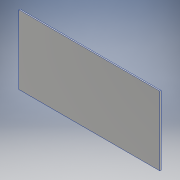
# Autodesk Inventor part: Led Plater
Saved by Autodesk Inventor 2017 (Build 210142000, 142)
## iProperties
Created: 2017-01-06
Part Number: Led Plater
Material: Aluminum 6061
Document SubType Name: Modeling
Designer: umr
Density: 2.7 g/cm^3
Appearance: Aluminum - Flat
Author: umr
Autodesk Inventor part; units mm, degrees
ref_plane "YZ Plane" through (0, 0, 0) normal (1, 0, 0) x (0, 1, 0)
sketch "Sketch1" plane through (0, 0, 0) normal (0, 1, 0) x (-1, 0, 0)
  line L0 (0, 0) -> (2550, 0)
  line L1 (2550, 0) -> (2550, -1250)
  line L2 (2550, -1250) -> (0, -1250)
  line L3 (0, -1250) -> (0, 0)
  dimension "d0" = 1250
  dimension "d1" = 2550
  constraints: 8 end point, 2 parallel, 1 horizontal, 1 perpendicular
  measures "d0" distance of L0.end L1.end
  measures "d1" distance between parallel lines of L3 L1
extrude "Extrusion1" add sketch "Sketch1" along normal blind 20
sketch "Sketch2" plane through (0, 20, 0) normal (0, 1, 0) x (1, 0, 0)
  line L0 (-2550, 0) -> (0, 0) projected
  line L1 (0, 0) -> (0, 1250) projected
  line L2 (0, 1250) -> (-2550, 1250) projected
  line L3 (-2550, 1250) -> (-2550, 0) projected
  circle A0 centre (-2500, 1100) radius 25
  dimension "d4" = 50
  dimension "d5" = 1250
  dimension "d6" = 150
  dimension "d7" = 50
  constraints: 1 centre point
  measures "d4" diameter of A0
  measures "d5" distance of L2.end L0.start
  measures "d6" distance from line of A0.centre L2
  measures "d7" distance from line of L3 A0.centre
ref_plane "Work Plane1" through (-1275, 0, -1250) normal (-1, 0, 0) x (0, 0, 1)
ref_plane "Work Plane2" through (0, 0, -625) normal (0, 0, -1) x (-1, 0, 0)
extrude "Extrusion2" cut sketch "Sketch2" against normal blind 10 contours A0
mirror "Mirror1" about plane through (0, 0, -625) normal (0, 0, -1) of "Extrusion2"
mirror "Mirror2" about plane through (-1275, 0, -1250) normal (-1, 0, 0) of "Extrusion2", "Mirror1"
body "Solid1"
